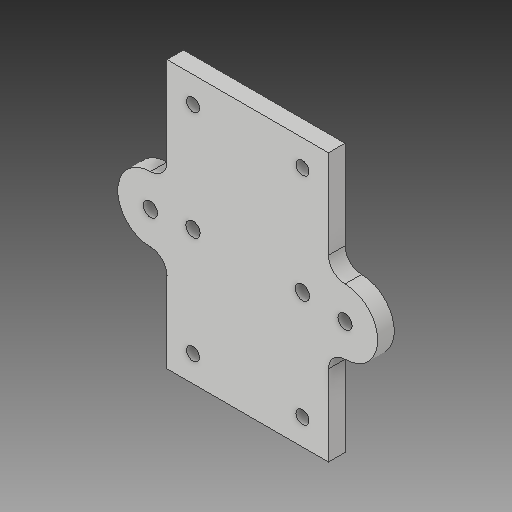
# Autodesk Inventor part: yCarraige
Saved by Autodesk Inventor 2019 (Build 230136000, 136)
## iProperties
Created: 2019-05-08
Part Number: yCarraige
Material: Generic
Document SubType Name: Modeling
Designer: Alex Jones
Density: 1 g/cm^3
Appearance: Default
Mass: 44.7415 g
Surface Area: 172.963 cm^2
Volume: 44.7415 cm^3
Author: Alex Jones
Autodesk Inventor part; units mm, degrees
ref_plane "YZ Plane" through (0, 0, 0) normal (1, 0, 0) x (0, 1, 0)
ref_plane "XZ Plane" through (0, 0, 0) normal (0, 1, 0) x (-1, 0, 0)
ref_plane "XY Plane" through (0, 0, 0) normal (0, 0, 1) x (1, 0, 0)
sketch "Sketch1" plane through (0, 0, 0) normal (0, 0, 1) x (1, 0, 0)
  circle A0 centre (-610.4613, 17.8) radius 2.5 projected
  circle A1 centre (-610.4613, 17.8) radius 9.9 construction
  circle A2 centre (-652.4613, 17.8) radius 2.5 projected
  circle A3 centre (-652.4613, 17.8) radius 9.9 construction
  circle A4 centre (-610.4613, -65) radius 2.5 projected
  circle A5 centre (-610.4613, -65) radius 9.9 construction
  circle A6 centre (-652.4613, -65) radius 2.5 projected
  circle A7 centre (-652.4613, -65) radius 9.9 construction
  line L0 (-610.4613, -65) -> (-652.4613, -65) construction
  line L1 (-652.4613, -65) -> (-652.4613, 17.8) construction
  line L2 (-652.4613, 17.8) -> (-610.4613, 17.8) construction
  line L3 (-610.4613, 17.8) -> (-610.4613, -65) construction
  line L4 (-662.4613, -75) -> (-600.4613, -75)
  line L5 (-600.4613, -75) -> (-600.4613, 27.8)
  line L6 (-600.4613, 27.8) -> (-662.4613, 27.8)
  line L7 (-662.4613, 27.8) -> (-662.4613, -75)
  point P0 (0, 0)
  dimension "d0" = 10
  constraints: 16 end point, 4 parallel, 2 perpendicular, 1 horizontal, 3 other
  measures "d0" distance between parallel lines of L0 L4
extrude "Extrusion1" add sketch "Sketch1" along normal blind 6.35
sketch "Sketch2" plane through (0, 0, 6.35) normal (0, 0, 1) x (1, 0, 0)
  circle A0 centre (-610.4613, 17.8) radius 2.5 projected
  circle A1 centre (-610.4613, -65) radius 2.5 projected
  circle A2 centre (-652.4613, -65) radius 2.5 projected
  circle A3 centre (-652.4613, 17.8) radius 2.5 projected
  circle A4 centre (-652.4613, 17.8) radius 2.5 projected
  line L0 (-652.4613, 17.8) -> (-652.4613, -65) construction
  circle A5 centre (-610.4613, 17.8) radius 2.5 projected
  circle A6 centre (-610.4613, -65) radius 2.5 projected
  line L1 (-610.4613, 17.8) -> (-610.4613, -65) construction
  circle A7 centre (-610.4613, -23.6) radius 2.75
  circle A8 centre (-652.4613, -23.6) radius 2.75
  point P0 (0, 0)
  dimension "d3" = 5.5
  constraints: 4 end point, 2 centre point, 2 midpoint, 2 vertical, 1 equal radius
  measures "d3" diameter of A8
extrude "Extrusion2" cut sketch "Sketch2" against normal blind 25.4 contours A7 | A8
sketch "Sketch3" plane through (0, 0, 6.35) normal (0, 0, 1) x (1, 0, 0)
  line L0 (-688.334, -23.6) -> (-567.3626, -23.6) construction
  line L1 (-600.4613, -75) -> (-600.4613, 27.8) construction
  line L2 (-662.4613, 27.8) -> (-662.4613, -75) construction
  line L3 (-594.1113, -75) -> (-594.1113, 27.8) construction
  line L4 (-668.8113, 24.7) -> (-668.8113, -75) construction
  circle A0 centre (-668.8113, -25.15) radius 2.75
  arc A1 (-668.8113, -12.6221) -> (-668.8113, -37.6779) centre (-668.8113, -25.15) ccw
  line L5 (-600.4613, -75) -> (-600.4613, 27.8) projected
  arc A2 (-662.4613, -44.0279) -> (-668.8113, -37.6779) centre (-668.8113, -44.0279) ccw
  arc A3 (-668.8113, -12.6221) -> (-662.4613, -6.2721) centre (-668.8113, -6.2721) ccw
  line L6 (-668.8113, -6.2721) -> (-662.4613, -6.2721) construction
  line L7 (-668.8113, -6.2721) -> (-668.8113, -12.6221) construction
  line L8 (-600.4613, 27.8) -> (-662.4613, 27.8) construction
  line L9 (-631.4613, 27.8) -> (-631.4613, -75) construction
  line L10 (-662.4613, -75) -> (-600.4613, -75) construction
  circle A4 centre (-594.1113, -25.15) radius 2.75
  arc A5 (-594.1113, -37.6779) -> (-594.1113, -12.6221) centre (-594.1113, -25.15) ccw
  arc A6 (-594.1113, -37.6779) -> (-600.4613, -44.0279) centre (-594.1113, -44.0279) ccw
  arc A7 (-600.4613, -6.2721) -> (-594.1113, -12.6221) centre (-594.1113, -6.2721) ccw
  line L11 (-594.1113, -6.2721) -> (-600.4613, -6.2721) construction
  line L12 (-594.1113, -6.2721) -> (-594.1113, -12.6221) construction
  line L13 (-662.4613, -6.2721) -> (-662.4613, -44.0279) construction
  line L14 (-662.4613, -6.2721) -> (-662.4613, -44.0279)
  line L15 (-600.4613, -44.0279) -> (-600.4613, -6.2721)
  point P0 (0, 0)
  point P1 (-574.5885, -23.6)
  dimension "d6" = 6.35
  dimension "d7" = 6.35
  dimension "d9" = 6.35
  dimension "d10" = 90
  dimension "d11" = 6.35
  dimension "d14" = 1.55
  dimension "d15" = 51.4
  constraints: 22 end point, 12 point on circle, 9 symmetric about line, 8 centre point, 4 point on line, 3 midpoint, 3 tangent, 2 coincident, 2 parallel, 1 collinear, 1 horizontal, 4 other
  measures "d6" distance between parallel lines of L2 L4
  measures "d7" distance between parallel lines of L1 L3
  measures "d9" radius of A2
  measures "d10" angle of L7 L6
  measures "d11" radius of A3
  measures "d14" distance from line of L0 A4.centre
  measures "d15" distance between parallel lines of L8 L0
extrude "Extrusion3" add sketch "Sketch3" against normal up to surface (6.35 mm away)
body "Solid1"
